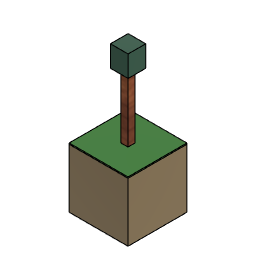
Tree without branches v1 (Autodesk Fusion 360 design; units mm, degrees)
Autodesk Fusion 360 part; units mm, degrees
note: some values were not read from the file. Chosen so that the rebuilt part matches the saved one: which face or edge a step refers to. Set by a fixed rule: which sketch regions a step uses.
sketch "Skizze1" plane through (0, 0, 0) normal (0, 0, 1) x (1, 0, 0)
  line L0 (0, 0) -> (50, 0)
  line L1 (50, 0) -> (50, 50)
  line L2 (50, 50) -> (0, 50)
  line L3 (0, 50) -> (0, 0)
  line L4 (0, 25) -> (50, 25) construction
  line L5 (25, 50) -> (25, 0) construction
  constraint coincident L0.start L3.end
  constraint midpoint L3 L4.start
  constraint midpoint L1 L4.end
  constraint midpoint L2 L5.start
  constraint midpoint L0 L5.end
  constraint perpendicular L0 L5
extrude "Extrusion1" add sketch "Skizze1" against normal blind 1 makes body 1 in component "Ground"
ref_plane "Arbeitsebene1" through (25, 25, 0) normal (0, -1, 0) x (1, 0, 0)
ref_plane "Arbeitsebene2" through (25, 25, 0) normal (-1, 0, 0) x (0, -1, 0)
sketch "Skizze2" plane through (25, 25, 0) normal (0, -1, 0) x (1, 0, 0)
  line L0 (-25, 0) -> (25, 0)
  line L1 (0, 0) -> (0, 75) construction
  line L2 (-3, 0) -> (-3, 64.4558)
  line L3 (-3, 64.4558) -> (3, 64.4558)
  line L4 (3, 64.4558) -> (3, 0)
  line L5 (-3, 0) -> (3, 0)
  line L6 (-4.6144, 10.8306) -> (-20.8773, 10.8306)
  line L7 (-20.8773, 10.8306) -> (-20.8773, 6.8306)
  line L8 (-20.8773, 6.8306) -> (-4.6144, 6.8306)
  line L9 (-4.6144, 6.8306) -> (-4.6144, 10.8306)
  line L10 (3, 44.9151) -> (20.4397, 44.9151)
  line L11 (20.4397, 44.9151) -> (20.4397, 40.9151)
  line L12 (20.4397, 40.9151) -> (3, 40.9151)
  line L13 (3, 40.9151) -> (3, 44.9151)
  line L14 (-24.5663, 15.2526) -> (-8.0379, 15.2526)
  line L15 (-8.0379, 15.2526) -> (-8.0379, 0.2526)
  line L16 (-8.0379, 0.2526) -> (-24.5663, 0.2526)
  line L17 (-24.5663, 0.2526) -> (-24.5663, 15.2526)
  line L18 (5.3079, 50.313) -> (22.7898, 50.313)
  line L19 (22.7898, 50.313) -> (22.7898, 35.313)
  line L20 (22.7898, 35.313) -> (5.3079, 35.313)
  line L21 (5.3079, 35.313) -> (5.3079, 50.313)
  line L22 (-7.4098, 73.036) -> (7.5902, 73.036)
  line L23 (7.5902, 73.036) -> (7.5902, 55)
  line L24 (7.5902, 55) -> (-7.4098, 55)
  line L25 (-7.4098, 55) -> (-7.4098, 73.036)
  dimension "d21" = 6
  dimension "d25" = 3
  dimension "d26" = 4
  dimension "d27" = 4
  dimension "d36" = 15
  dimension "d37" = 15
  dimension "d38" = 15
  constraint coincident L1.start origin
  constraint perpendicular L0 L1
  constraint coincident L0 L2.start
  constraint perpendicular L0 L2
  constraint perpendicular L1 L3
  constraint coincident L0 L4.end
  constraint perpendicular L0 L4
  constraint horizontal L6
  constraint vertical L7
  constraint horizontal L8
  constraint horizontal L10
  constraint vertical L11
  constraint horizontal L12
  constraint vertical L13
  constraint coincident L4 L10.start
  constraint horizontal L14
  constraint vertical L15
  constraint horizontal L16
  constraint vertical L17
  constraint horizontal L18
  constraint vertical L19
  constraint horizontal L20
  constraint vertical L21
  constraint horizontal L22
  constraint vertical L23
  constraint horizontal L24
  constraint vertical L25
  constraint perpendicular L6 L9
  measures "d21" distance of L2.end L3.end
  measures "d25" distance of L1 L2
  measures "d26" distance of L6 L8
  measures "d27" distance of L10.end L11.end
  measures "d36" distance of L18.end L19.end
  measures "d37" distance of L14.start L16.end
  measures "d38" distance of L22.start L22.end
extrude "Extrusion1'" add sketch "Skizze2" along normal mid plane 6 separate body contours L0 L2 L4 L5 L13 L24 | L2 L3 L4 L24 makes body 2 in component "Trunk"
sketch "Skizze3" plane through (25, 25, 0) normal (-1, 0, 0) x (0, 1, 0)
  line L0 (3, -64.4558) -> (-3, -64.4558)
  line L1 (-3, -64.4558) -> (-3, 0)
  line L2 (-3, 0) -> (3, 0)
  line L3 (3, 0) -> (3, -64.4558)
  line L4 (0, -44.9151) -> (0, -40.9151)
  line L5 (0, -10.8306) -> (0, -6.8306)
  line L6 (3, -40.2798) -> (19.6821, -40.2798)
  line L7 (19.6821, -40.2798) -> (19.6821, -36.2798)
  line L8 (19.6821, -36.2798) -> (3, -36.2798)
  line L9 (3, -36.2798) -> (3, -40.2798)
  line L10 (-5.1445, -8.9762) -> (-20.0951, -8.9762)
  line L11 (-20.0951, -8.9762) -> (-20.0951, -4.9762)
  line L12 (-20.0951, -4.9762) -> (-5.1445, -4.9762)
  line L13 (8.1625, -45.8226) -> (23.7982, -45.8226)
  line L14 (23.7982, -45.8226) -> (23.7982, -30.8226)
  line L15 (23.7982, -30.8226) -> (8.1625, -30.8226)
  line L16 (8.1625, -30.8226) -> (8.1625, -45.8226)
  line L17 (-24.6875, -14.8967) -> (-8.5018, -14.8967)
  line L18 (-8.5018, -14.8967) -> (-8.5018, 0.1033)
  line L19 (-8.5018, 0.1033) -> (-24.6875, 0.1033)
  line L20 (-24.6875, 0.1033) -> (-24.6875, -14.8967)
  line L21 (-20.0951, -6.9762) -> (-5.1445, -6.9762) construction
  line L22 (3, -38.2798) -> (19.6821, -38.2798) construction
  line L23 (-5.1445, -8.9762) -> (-5.1445, -4.9762)
  dimension "d32" = 4
  dimension "d33" = 4
  dimension "d34" = 15
  dimension "d35" = 15
  constraint horizontal L6
  constraint vertical L7
  constraint horizontal L8
  constraint vertical L9
  constraint coincident L3 L6.start
  constraint horizontal L10
  constraint vertical L11
  constraint horizontal L12
  constraint horizontal L13
  constraint vertical L14
  constraint horizontal L15
  constraint vertical L16
  constraint horizontal L17
  constraint vertical L18
  constraint horizontal L19
  constraint vertical L20
  constraint midpoint L11 L21.start
  constraint midpoint L9 L22.start
  constraint midpoint L7 L22.end
  constraint perpendicular L10 L23
  constraint midpoint L21.end L23
  measures "d32" distance of L10.end L11.end
  measures "d33" distance of L6.end L7.end
  measures "d34" distance of L17 L19
  measures "d35" distance of L13 L15
extrude "Extrusion1''" add sketch "Skizze3" along normal mid plane 4 separate body contours L3 L6 L8 L9 L16 | L6 L7 L8 L16 | L10 L12 L18 L23 | L10 L11 L12 L18 makes body 3 at (23, 14.872, 7.6428) makes body 4 at (23, 39.1214, 38.9465) in component "Branches Y"
extrude "Extrusion1'''" add sketch "Skizze2" along normal mid plane 4 separate body contours L4 L10 L12 L13 L21 | L10 L11 L12 L21 | L6 L8 L9 L15 | L6 L7 L8 L15 makes body 5 at (14.9646, 23, 9.4973) makes body 6 at (33.8132, 23, 42.2484) in component "Branches X"
extrude "Extrusion1''''" add sketch "Skizze2" along normal mid plane 15 separate body contours L2 L3 L4 L22 L23 L24 L25 | L2 L3 L4 L24 | L10 L11 L12 L21 | L10 L11 L12 L18 L19 L20 L21 | L6 L7 L8 L15 | L6 L7 L8 L14 L15 L16 L17 makes body 7 at (5.9431, 17.5, 10.2526) makes body 8 at (36.1352, 17.5, 45.313) makes body 9 at (17.5902, 27.5, 61.012) in component "Leaf X"
extrude "Extrusion1'''''" add sketch "Skizze3" along normal mid plane 15 separate body contours L6 L7 L8 L16 | L6 L7 L8 L13 L14 L15 L16 | L10 L11 L12 L17 L18 L19 L20 | L10 L11 L12 L18 makes body 10 at (27.5, 5.7077, 14.8967) makes body 11 at (17.5, 38.3744, 35.8226) in component "Leaf Y"
extrude "Extrusion1''''''" add 1 faces at (16.6667, 33.3333, -1) along direction (0, 0, -1) blind 50 separate body on bodies 1 makes body 12 in component "Ground below"
component "Ground" placed x (1, 0, 0) y (0, 1, 0) z (0, 0, 1) at (0, 0, 0)
component "Trunk" placed x (1, 0, 0) y (0, 1, 0) z (0, 0, 1) at (0, 0, 0)
component "Branches Y" placed x (1, 0, 0) y (0, 1, 0) z (0, 0, 1) at (0, 0, 0)
component "Branches X" placed x (1, 0, 0) y (0, 1, 0) z (0, 0, 1) at (0, 0, 0)
component "Leaf X" placed x (1, 0, 0) y (0, 1, 0) z (0, 0, 1) at (0, 0, 0)
component "Leaf Y" placed x (1, 0, 0) y (0, 1, 0) z (0, 0, 1) at (0, 0, 0)
component "Ground below" placed x (1, 0, 0) y (0, 1, 0) z (0, 0, 1) at (0, 0, 0)
hidden bodies 7 8
equation "d21 = d_trunk"
equation "d_trunk = 6 mm" comment "Diameter Treetrunk"
equation "d_branch = 4 mm" comment "Diameter tree branch"
equation "d_leaf = 15 mm" comment "diameter leafball"
equation "d25 = d21 / 2"
equation "d26 = d_branch"
equation "d27 = d_branch"
equation "d30 = d_trunk / 2"
equation "d32 = d_branch"
equation "d33 = d_branch"
equation "d34 = d_leaf"
equation "d35 = d_leaf"
equation "d36 = d_leaf"
equation "d37 = d_leaf"
equation "d38 = d_leaf"
equation "d39 = d_branch / 2"
equation "d41 = d_branch / 2"
equation "d43 = d_leaf / 2"
equation "d45 = d_leaf / 2"
